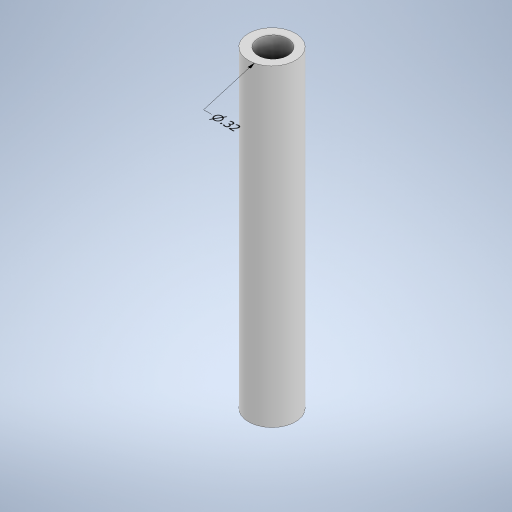
# Autodesk Inventor part: Central_Rotator
Saved by Autodesk Inventor 2024 (Build 280153000, 153)
## iProperties
Created: 2025-01-23
Part Number: Central_Rotator
Material: Generic
Document SubType Name: Modeling
Designer: b_arm
Density: 1 g/cm^3
Appearance: Default
Author: b_arm
## iProperties of the stored document central rotator claw grabber_3DPrint.ipt
Created: 2025-02-18
Part Number: central rotator claw grabber_3DPrint
Material: Generic
Document SubType Name: Modeling
Designer: b_arm
Density: 1 g/cm^3
Appearance: Default
Author: b_arm
Autodesk Inventor part; units mm, degrees
ref_plane "YZ Plane" through (0, 0, 0) normal (1, 0, 0) x (0, 1, 0)
ref_plane "XZ Plane" through (0, 0, 0) normal (0, 1, 0) x (-1, 0, 0)
sketch "Sketch1" plane through (0, 0, 0) normal (0, 1, 0) x (-1, 0, 0)
  circle A0 centre (0, 0) radius 4.0005
  dimension "d0" = 8.001
  constraints: 1 centre point, 1 coincident
  measures "d0" diameter of A0
extrude "Extrusion1" add sketch "Sketch1" along normal blind 53.34
ref_plane "Work Plane1" through (0, 26.67, 0) normal (0, -1, 0) x (1, 0, 0)
sketch "Sketch3" plane through (0, 0, 0) normal (0, -1, 0) x (1, 0, 0)
  point P0 (0, 0)
  point P1 (-0.1045, -0.2801)
hole "Hole1" at (-0.1045, 0, -0.2801) direction (0, 1, 0) diameter 5.08 depth 11.0363
sketch "Sketch4" plane through (0, 53.34, 0) normal (0, 1, 0) x (1, 0, 0)
  point P0 (0, 0)
  point P1 (0.1091, 0.0558)
hole "Hole2" at (0.1091, 53.34, -0.0558) direction (0, -1, 0) diameter 5.08 depth 11.0363
body "Solid1"
